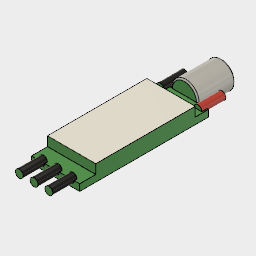
DYS ESC BL40 v2 (Autodesk Fusion 360 design; units mm, degrees)
Autodesk Fusion 360 part; units mm, degrees
note: some values were not read from the file. Set by a fixed rule: which sketch regions a step uses.
sketch "Sketch1" plane through (0, 0, 0) normal (0, 1, 0) x (1, 0, 0)
  line L0 (-9, 24) -> (9, 24)
  line L1 (9, 24) -> (9, -24)
  line L2 (9, -24) -> (-9, -24)
  line L3 (-9, -24) -> (-9, 24)
  line L4 (-9, 24) -> (9, -24) construction
  line L5 (9, 24) -> (-9, -24) construction
  dimension "d1" = 18
  dimension "d2" = 48
  measures "d1" distance of L1.end L2.end
  measures "d2" distance of L0.end L1.end
extrude "Extrude1" add sketch "Sketch1" against normal blind 2.5
sketch "Sketch2" plane through (0, 0, 0) normal (0, 1, 0) x (-1, 0, 0)
  line L0 (9, 24) -> (-9, 24)
  line L1 (-9, 24) -> (-9, -24)
  line L2 (-9, -24) -> (9, -24)
  line L3 (9, -24) -> (9, 24)
  line L4 (9, -19) -> (-9, -19)
  line L5 (-9, -19) -> (-9, 18)
  line L6 (-9, 18) -> (9, 18)
  line L7 (9, 18) -> (9, -19)
  dimension "d5" = 37
  dimension "d6" = 5
  measures "d5" distance of L4.end L5.end
  measures "d6" distance of L2 L4
extrude "Extrude2" add sketch "Sketch2" along normal blind 3.5 contours L1 L3 L4 L5 L6 L7
sketch "Sketch3" plane through (0, 0, -24) normal (0, 0, -1) x (-1, 0, 0)
  line L0 (9, 0) -> (-9, 0)
  line L1 (-9, 0) -> (-9, -2.5)
  line L2 (-9, -2.5) -> (9, -2.5)
  line L3 (9, -2.5) -> (9, 0)
  circle A0 centre (0, 0) radius 5
  dimension "d9" = 10
  measures "d9" diameter of A0
extrude "Extrude3" add sketch "Sketch3" along normal blind 14 contours L0 L2 A0 | L0 A0 | L2 A0
fillet "Fillet1" radius 0.5 5 edges at (4.6616, -1.8081, -38) (0, 5, -24) (4.8296, -1.2941, -24) (0, -5, -24) (-4.8296, -1.2941, -24)
sketch "Sketch4" plane through (0, 0, 24) normal (0, 0, 1) x (1, 0, 0)
  line L0 (9, 0) -> (-9, 0)
  line L1 (-9, 0) -> (-9, -2.5)
  line L2 (-9, -2.5) -> (9, -2.5)
  line L3 (9, -2.5) -> (9, 0)
  circle A0 centre (0, 0) radius 1.5
  circle A1 centre (5.5, 0) radius 1.5
  circle A2 centre (-5.5, 0) radius 1.5
  point P0 (5.5, 0)
  point P1 (-5.5, 0)
  dimension "d13" = 3
  measures "d13" diameter of A0
extrude "Extrude4" add sketch "Sketch4" along normal blind 8 contours L0 A1 | L0 A1 | L0 A0 | L0 A0 | L0 A2 | L0 A2
extrude "Extrude5" add 3 faces at (5.8665, 0.3401, 24) (0.3665, 0.3401, 24) (-5.1335, 0.3401, 24) along direction (0, 0, -1) blind 1
sketch "Sketch5" plane through (0, 0, -24) normal (0, 0, -1) x (-1, 0, 0)
  arc A0 (-5.5, 0) -> (-4.899, -2.5) centre (0, 0) ccw
  line L0 (-5.5, 0) -> (-9, 0)
  line L1 (-9, 0) -> (-9, -2.5)
  line L2 (-9, -2.5) -> (-4.899, -2.5)
  circle A1 centre (-7, 0) radius 1.5
  circle A2 centre (7, 0) radius 1.5
  point P0 (-7, 0)
  point P1 (7, 0)
  dimension "d18" = 3
  dimension "d19" = 3
  measures "d18" diameter of A1
  measures "d19" diameter of A2
extrude "Extrude6" add sketch "Sketch5" along normal blind 7 contours L0 A1 | L0 A1 | A2
extrude "Extrude7" add 2 faces at (-7.3665, 0.4891, -24) (6.6335, 0.3401, -24) along direction (0, 0, 1) blind 2
